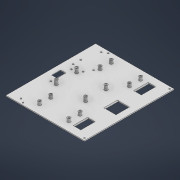
# Autodesk Inventor part: Obenplatte_hinten
Saved by Autodesk Inventor 2021 (Build 250183000, 183)
## iProperties
Created: 2021-02-01
Part Number: Obenplatte_hinten
Material: Generisch
Document SubType Name: Modeling
Designer: laure
Density: 1 g/cm^3
Appearance: Vorgabe
Author: laure
## iProperties of the stored document _3D-Druck.ipt
Created: 2021-02-04
Part Number: _3D-Druck
Material: Generisch
Document SubType Name: Modeling
Designer: Ctroi
Density: 1 g/cm^3
Appearance: Vorgabe
Author: Ctroi
Autodesk Inventor part; units mm, degrees
ref_plane "YZ Plane" through (0, 0, 0) normal (1, 0, 0) x (0, 1, 0)
ref_plane "XZ Plane" through (0, 0, 0) normal (0, 1, 0) x (-1, 0, 0)
ref_plane "XY Plane" through (0, 0, 0) normal (0, 0, 1) x (1, 0, 0)
sketch "Skizze1" plane through (0, 0, 0) normal (0, 1, 0) x (-1, 0, 0)
  line L0 (87.5, -100) -> (-87.5, -100)
  line L1 (-87.5, -100) -> (-87.5, 100)
  line L2 (-87.5, 100) -> (87.5, 100)
  line L3 (87.5, 100) -> (87.5, -100)
  line L4 (0, -140) -> (0, 140) projected
  line L5 (-122.5, 0) -> (122.5, 0) projected
  point P0 (0, 0)
  dimension "d0" = 175
  dimension "d1" = 200
  constraints: 8 end point, 2 parallel, 1 horizontal, 1 perpendicular, 2 other
  measures "d0" distance of L1.end L2.end
  measures "d1" distance of L0.end L1.end
extrude "Extrusion1" add sketch "Skizze1" along normal blind 2
sketch "Skizze2" plane through (0, 2, 0) normal (0, 1, 0) x (1, 0, 0)
  circle A0 centre (-54.5, 95) radius 1.6
  line L0 (0, 140) -> (0, -140) projected
  line L1 (122.5, 0) -> (-122.5, 0) projected
  line L2 (87.5, 100) -> (-87.5, 100) projected
  circle A1 centre (82.5, 95) radius 1.6
  circle A2 centre (-54.5, -95) radius 1.6
  circle A3 centre (82.5, -95) radius 1.6
  line L3 (-87.5, 100) -> (-87.5, -100) projected
  line L4 (87.5, -100) -> (87.5, 100) projected
  point P0 (0, 0)
  dimension "d4" = 3.2
  dimension "d6" = 5
  dimension "d7" = 3.2
  dimension "d9" = 5
  dimension "d40" = 33
  dimension "d41" = 5
  constraints: 4 centre point, 2 symmetric about line, 2 other
  measures "d4" diameter of A0
  measures "d6" distance from line of A0.centre L2
  measures "d7" diameter of A1
  measures "d9" distance from line of L2 A1.centre
  measures "d40" distance from line of L3 A0.centre
  measures "d41" distance from line of L4 A1.centre
extrude "Extrusion2" cut sketch "Skizze2" against normal up to surface (2 mm away) contours A0 | A1 | A2 | A3
sketch "Skizze3" plane through (0, 2, 0) normal (0, 1, 0) x (1, 0, 0)
  line L0 (87.5, -100) -> (87.5, 100) projected
  line L1 (-87.5, -100) -> (87.5, -100) projected
  line L2 (87.5, 100) -> (-87.5, 100) projected
  circle A0 centre (-64.5, 89.5) radius 1.6
  line L3 (-87.5, 100) -> (-87.5, -100) projected
  circle A1 centre (-64.5, 23) radius 1.6
  circle A2 centre (-64.5, -23) radius 1.6
  circle A3 centre (-64.5, -89.5) radius 1.6
  point P0 (0, 0)
  dimension "d26" = 3.2
  dimension "d27" = 23
  dimension "d28" = 10.5
  dimension "d29" = 3.2
  dimension "d30" = 23
  dimension "d31" = 77
  dimension "d32" = 3.2
  dimension "d33" = 23
  dimension "d34" = 77
  dimension "d35" = 3.2
  dimension "d36" = 10.5
  dimension "d37" = 23
  constraints: 4 centre point
  measures "d26" diameter of A0
  measures "d27" distance from line of L3 A0.centre
  measures "d28" distance from line of L2 A0.centre
  measures "d29" diameter of A1
  measures "d30" distance from line of L3 A1.centre
  measures "d31" distance from line of L2 A1.centre
  measures "d32" diameter of A2
  measures "d33" distance from line of L3 A2.centre
  measures "d34" distance from line of L1 A2.centre
  measures "d35" diameter of A3
  measures "d36" distance from line of L1 A3.centre
  measures "d37" distance from line of L3 A3.centre
extrude "Extrusion4" cut sketch "Skizze3" against normal up to surface (2 mm away) contours A0 | A1 | A2 | A3
sketch "Skizze4" plane through (0, 2, 0) normal (0, 1, 0) x (1, 0, 0)
  line L0 (-75.5, -10) -> (-65.5, -10)
  line L1 (-65.5, -10) -> (-65.5, 10)
  line L2 (-65.5, 10) -> (-75.5, 10)
  line L3 (-75.5, 10) -> (-75.5, -10)
  line L4 (-75.5, -10) -> (-65.5, 10) construction
  line L5 (-65.5, -10) -> (-75.5, 10) construction
  line L6 (-87.5, 100) -> (-87.5, -100) projected
  line L7 (87.5, 100) -> (-87.5, 100) projected
  point P0 (0, 0)
  point P1 (-70.5, 0)
  dimension "d42" = 10
  dimension "d43" = 20
  dimension "d44" = 12
  dimension "d45" = 90
  constraints: 12 end point, 2 midpoint, 2 parallel, 1 horizontal, 1 perpendicular
  measures "d42" distance of L2.end L1.end
  measures "d43" distance of L1.end L0.end
  measures "d44" distance between parallel lines of L6 L3
  measures "d45" distance between parallel lines of L7 L2
extrude "Extrusion5" cut sketch "Skizze4" against normal up to surface (2 mm away)
fillet "Rundung1" radius 2 1 edges at (-75.5, 0, 0)
fillet "Rundung2" radius 2 1 edges at (-65.5, 2, 0)
sketch "Skizze5" plane through (0, 2, 0) normal (0, 1, 0) x (1, 0, 0)
  circle A0 centre (-32.5, 80) radius 3.5
  circle A1 centre (33, 80) radius 3.5
  circle A2 centre (-32.5, 55) radius 3.5
  circle A3 centre (33, 55) radius 3.5
  line L0 (87.5, 100) -> (-87.5, 100) projected
  line L1 (-87.5, 100) -> (-87.5, -100) projected
  line L2 (48, 83.5) -> (63, 83.5)
  line L3 (63, 83.5) -> (63, 51.5)
  line L4 (63, 51.5) -> (48, 51.5)
  line L5 (48, 51.5) -> (48, 83.5)
  line L6 (122.5, 0) -> (-122.5, 0) projected
  circle A4 centre (-32.5, -80) radius 3.5
  circle A5 centre (33, -80) radius 3.5
  circle A6 centre (-32.5, -55) radius 3.5
  circle A7 centre (33, -55) radius 3.5
  line L7 (48, -83.5) -> (63, -83.5)
  line L8 (63, -83.5) -> (63, -51.5)
  line L9 (63, -51.5) -> (48, -51.5)
  line L10 (48, -51.5) -> (48, -83.5)
  circle A8 centre (-52.5, 22.75) radius 3.5
  circle A9 centre (-52.5, -22.75) radius 3.5
  circle A10 centre (13, 22.75) radius 3.5
  circle A11 centre (13, -22.75) radius 3.5
  line L11 (48, 15) -> (73, 15)
  line L12 (73, 15) -> (73, -15)
  line L13 (73, -15) -> (48, -15)
  line L14 (48, -15) -> (48, 15)
  line L15 (87.5, -100) -> (87.5, 100) projected
  point P0 (0, 0)
  dimension "d50" = 7
  dimension "d51" = 7
  dimension "d52" = 7
  dimension "d53" = 7
  dimension "d54" = 20
  dimension "d55" = 20
  dimension "d56" = 55
  dimension "d57" = 65.5
  dimension "d58" = 55
  dimension "d59" = 65.5
  dimension "d60" = 25
  dimension "d61" = 25
  dimension "d62" = 15
  dimension "d63" = 15
  dimension "d64" = 16.5
  dimension "d65" = 32
  dimension "d81" = 7
  dimension "d82" = 7
  dimension "d83" = 7
  dimension "d84" = 7
  dimension "d85" = 35
  dimension "d86" = 35
  dimension "d87" = 45.5
  dimension "d88" = 45.5
  dimension "d89" = 22.75
  dimension "d90" = 22.75
  dimension "d91" = 65.5
  dimension "d92" = 65.5
  dimension "d93" = 25
  dimension "d94" = 30
  dimension "d95" = 14.5
  constraints: 24 end point, 12 centre point, 8 symmetric about line, 4 parallel, 2 horizontal, 2 perpendicular, 5 other
  measures "d50" diameter of A0
  measures "d51" diameter of A1
  measures "d52" diameter of A2
  measures "d53" diameter of A3
  measures "d54" distance from line of L0 A0.centre
  measures "d55" distance from line of L0 A1.centre
  measures "d56" distance from line of L1 A0.centre
  measures "d57" distance of A0.centre A1.centre
  measures "d58" distance from line of L1 A2.centre
  measures "d59" distance of A2.centre A3.centre
  measures "d60" distance of A0.centre A2.centre
  measures "d61" distance of A1.centre A3.centre
  measures "d62" distance of L3.end L4.end
  measures "d63" distance from line of A1.centre L5
  measures "d64" distance between parallel lines of L0 L2
  measures "d65" distance between parallel lines of L2 L4
  measures "d81" diameter of A8
  measures "d82" diameter of A9
  measures "d83" diameter of A10
  measures "d84" diameter of A11
  measures "d85" distance from line of L1 A9.centre
  measures "d86" distance from line of L1 A8.centre
  measures "d87" distance of A8.centre A9.centre
  measures "d88" distance of A10.centre A11.centre
  measures "d89" distance from line of L6 A10.centre
  measures "d90" distance from line of L6 A8.centre
  measures "d91" distance of A10.centre A8.centre
  measures "d92" distance of A9.centre A11.centre
  measures "d93" distance of L12.end L13.end
  measures "d94" distance of L11.end L12.end
  measures "d95" distance between parallel lines of L15 L12
extrude "Extrusion6" add sketch "Skizze5" along normal blind 7 contours A0 | A1 | A2 | A3 | A4 | A5 | A6 | A7
extrude "Extrusion8" cut sketch "Skizze5" against normal up to surface (2 mm away) contours L12 L13 L14 L6 | L6 L14 L11 L12 | L2 L3 L4 L5 | L10 L9 L8 L7
fillet "Rundung3" radius 2 3 edges at (48, 2, -67.5) (48, 2, 67.5) (48, 2, 0)
extrude "Extrusion9" add sketch "Skizze5" along normal blind 10 contours A8 | A9 | A10 | A11
sketch "Skizze6" plane through (-32.5, 9, -80) normal (0, 1, 0) x (1, 0, 0)
  circle A0 centre (0, 0) radius 3.5 projected
  circle A1 centre (0, -25) radius 3.5 projected
  circle A2 centre (65.5, -25) radius 3.5 projected
  circle A3 centre (65.5, 0) radius 3.5 projected
  circle A4 centre (65.5, -135) radius 3.5 projected
  circle A5 centre (65.5, -160) radius 3.5 projected
  circle A6 centre (0, -160) radius 3.5 projected
  circle A7 centre (0, -135) radius 3.5 projected
  circle A8 centre (0, 0) radius 2
  circle A9 centre (0, -25) radius 2
  circle A10 centre (65.5, -25) radius 2
  circle A11 centre (65.5, 0) radius 2
  circle A12 centre (0, -135) radius 3.5 projected
  circle A13 centre (0, -135) radius 2
  circle A14 centre (0, -160) radius 2
  circle A15 centre (65.5, -135) radius 3.5 projected
  circle A16 centre (65.5, -135) radius 2
  circle A17 centre (65.5, -160) radius 2
  point P0 (32.5, -80)
  dimension "d68" = 4
  dimension "d69" = 4
  dimension "d70" = 4
  dimension "d71" = 4
  dimension "d72" = 4
  dimension "d73" = 4
  dimension "d74" = 4
  dimension "d75" = 4
  constraints: 8 centre point, 8 coincident
  measures "d68" diameter of A8
  measures "d69" diameter of A9
  measures "d70" diameter of A10
  measures "d71" diameter of A11
  measures "d72" diameter of A13
  measures "d73" diameter of A14
  measures "d74" diameter of A16
  measures "d75" diameter of A17
extrude "Extrusion7" cut sketch "Skizze6" against normal blind 5 contours A8 | A9 | A10 | A11 | A13 | A14 | A16 | A17
sketch "Skizze8" plane through (-52.5, 12, -22.75) normal (0, 1, 0) x (1, 0, 0)
  circle A0 centre (0, 0) radius 3.5 projected
  circle A1 centre (65.5, 0) radius 3.5 projected
  circle A2 centre (65.5, -45.5) radius 3.5 projected
  circle A3 centre (0, -45.5) radius 3.5 projected
  circle A4 centre (0, 0) radius 3.5 projected
  circle A5 centre (0, 0) radius 2
  circle A6 centre (65.5, 0) radius 3.5 projected
  circle A7 centre (65.5, 0) radius 2
  circle A8 centre (65.5, -45.5) radius 3.5 projected
  circle A9 centre (65.5, -45.5) radius 2
  circle A10 centre (0, -45.5) radius 3.5 projected
  circle A11 centre (0, -45.5) radius 2
  point P0 (52.5, -22.75)
  dimension "d98" = 4
  dimension "d99" = 4
  dimension "d100" = 4
  dimension "d101" = 4
  constraints: 4 centre point, 4 coincident
  measures "d98" diameter of A5
  measures "d99" diameter of A7
  measures "d100" diameter of A9
  measures "d101" diameter of A11
extrude "Extrusion10" cut sketch "Skizze8" against normal blind 5 contours A5 | A7 | A9 | A11
sketch "Skizze9" plane through (0, 2, 0) normal (0, 1, 0) x (1, 0, 0)
  circle A0 centre (-52.5, 22.75) radius 2 projected
  circle A1 centre (-32.5, 55) radius 2 projected
  line L0 (-52.5, 22.75) -> (-32.5, 55)
  circle A2 centre (-46.9798, 31.6513) radius 1.6
  circle A3 centre (-38.0202, 46.0987) radius 1.6
  circle A4 centre (-42.5, 38.875) radius 0.1
  circle A5 centre (-72.5, 52) radius 1.6
  circle A6 centre (-72.5, 35) radius 1.6
  line L1 (-87.5, 100) -> (-87.5, -100) projected
  line L2 (122.5, 0) -> (-122.5, 0) projected
  point P0 (0, 0)
  dimension "d104" = 3.2
  dimension "d105" = 3.2
  dimension "d106" = 13.8
  dimension "d107" = 0.2
  dimension "d108" = 6.8
  dimension "d109" = 3.2
  dimension "d110" = 3.2
  dimension "d111" = 15
  dimension "d112" = 15
  dimension "d113" = 17
  dimension "d114" = 35
  constraints: 5 centre point, 2 end point, 2 point on line, 1 coincident, 1 midpoint
  measures "d104" diameter of A2
  measures "d105" diameter of A3
  measures "d107" diameter of A4
  measures "d109" diameter of A5
  measures "d110" diameter of A6
  measures "d111" distance from line of L1 A6.centre
  measures "d112" distance from line of L1 A5.centre
  measures "d113" distance of A5.centre A6.centre
  measures "d114" distance from line of L2 A6.centre
extrude "Extrusion11" cut sketch "Skizze9" against normal up to surface (2 mm away) contours A2 L0 | L0 A2 | A3 L0 | L0 A3 | A5 | A6
